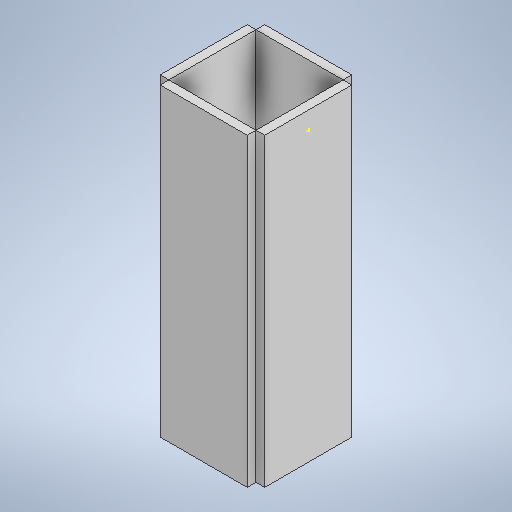
# Autodesk Inventor part: Landing Holder
Saved by Autodesk Inventor 2025.3 (Build 293356000, 356)
## iProperties
Created: 2026-04-19
Part Number: Landing Holder
Material: Generic
Document SubType Name: Modeling
Designer: kamal
Density: 1 g/cm^3
Appearance: Default
Author: kamal
Autodesk Inventor part; units mm, degrees
ref_plane "YZ Plane" through (0, 0, 0) normal (1, 0, 0) x (0, 1, 0)
ref_plane "XZ Plane" through (0, 0, 0) normal (0, 1, 0) x (-1, 0, 0)
ref_plane "XY Plane" through (0, 0, 0) normal (0, 0, 1) x (1, 0, 0)
sketch "Sketch1" plane through (0, 0, 0) normal (0, 1, 0) x (-1, 0, 0)
  line L0 (-20, -20) -> (20, -20)
  line L1 (20, -20) -> (20, 20)
  line L2 (20, 20) -> (-20, 20)
  line L3 (-20, 20) -> (-20, -20)
  line L4 (-20, -20) -> (20, 20) construction
  line L5 (20, -20) -> (-20, 20) construction
  line L6 (30, 30) -> (30, -30)
  line L7 (30, -30) -> (-30, -30)
  line L8 (-30, -30) -> (-30, 30)
  line L9 (-30, 30) -> (30, 30)
  line L10 (-25, 25) -> (25, 25)
  line L11 (25, 25) -> (25, -25)
  line L12 (25, -25) -> (-25, -25)
  line L13 (-25, -25) -> (-25, 25)
  line L14 (25, 25) -> (25, 30)
  line L15 (25, 25) -> (30, 25)
  line L16 (-25, 25) -> (-25, 30)
  line L17 (-25, 25) -> (-30, 25)
  line L18 (-25, -25) -> (-30, -25)
  line L19 (-25, -25) -> (-25, -30)
  line L20 (25, -25) -> (30, -25)
  line L21 (25, -25) -> (25, -30)
  line L22 (0, 25) -> (0, 30)
  line L23 (0, -25) -> (0, -30)
  point P0 (0, 0)
  dimension "d0" = 40
  dimension "d1" = 40
  dimension "d2" = 10
  dimension "d3" = 5
  constraints: 48 end point, 10 point on line, 9 perpendicular, 6 midpoint, 6 parallel, 1 horizontal, 6 other
  measures "d0" distance of L2.end L1.end
  measures "d1" distance of L1.end L0.end
  measures "d2" distance between parallel lines of L1 L6
  measures "d3" distance between parallel lines of L2 L10
extrude "Extrusion1" add sketch "Sketch1" along normal blind 10 contours L6 L20 L11 L15 | L14 L10 L22 L9 | L22 L10 L16 L9 | L21 L7 L23 L12 | L23 L7 L19 L12 | L13 L18 L8 L17
extrude "Extrusion2" add sketch "Sketch1" against normal blind 165 contours L6 L20 L11 L15 | L14 L10 L22 L9 | L22 L10 L16 L9 | L21 L7 L23 L12 | L23 L7 L19 L12 | L13 L18 L8 L17
sketch "Sketch2" plane through (30, 10, 25) normal (1, 0, 0) x (0, 0, -1)
  point P0 (25, -10)
body "Solid1"
